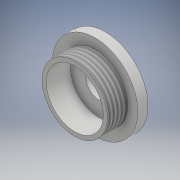
# Autodesk Inventor part: LagerDeckel
Saved by Autodesk Inventor 2017 (Build 210142000, 142)
## iProperties
Created: 2019-06-21
Part Number: LagerDeckel
Material: Generic
Document SubType Name: Modeling
Designer: Ole Simmering
Density: 1 g/cm^3
Appearance: Default
Author: Ole Simmering
Autodesk Inventor part; units mm, degrees
ref_plane "YZ Plane" through (0, 0, 0) normal (1, 0, 0) x (0, 1, 0)
ref_plane "XZ Plane" through (0, 0, 0) normal (0, 1, 0) x (-1, 0, 0)
ref_plane "XY Plane" through (0, 0, 0) normal (0, 0, 1) x (1, 0, 0)
sketch "Sketch1" plane through (0, 0, 0) normal (0, 0, 1) x (1, 0, 0)
  line L0 (0, 0) -> (0, 13.3519) construction
  line L1 (14, -12) -> (14, 0)
  line L2 (14, 0) -> (6.5, 0)
  line L3 (6.5, 3) -> (21, 3)
  line L4 (21, 3) -> (21, -2)
  line L5 (21, -2) -> (16, -2)
  line L6 (16, -2) -> (16, -12)
  line L7 (16, -12) -> (14, -12)
  line L8 (6.5, 3) -> (6.5, 0)
  line L9 (0, 0) -> (6.5, 0) construction
  dimension "d0" = 28
  dimension "d1" = 12
  dimension "d2" = 10
  dimension "d3" = 32
  dimension "d4" = 5
  dimension "d5" = 42
  dimension "d9" = 13
  constraints: 20 end point, 5 perpendicular, 2 horizontal, 2 vertical
  measures "d0" diameter of L1 L0
  measures "d1" distance of L1.start L1.end
  measures "d2" distance of L5.end L6.end
  measures "d3" diameter of L6 L0
  measures "d4" distance of L3.end L4.end
  measures "d5" diameter of L4 L0
  measures "d9" diameter of L8 L0
revolve "Revolution1" add sketch "Sketch1" angle 360 about axis through (0, 0, 0) along (0, 1, 0)
thread "Thread1" size "M32x2" class "6g" standard "ANSI Metric M Profile" full length
body "Solid1"
